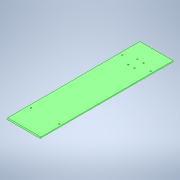
# Autodesk Inventor part: 前カバー中盤
Saved by Autodesk Inventor 2022 (Build 260153000, 153)
## iProperties
Created: 2022-11-07
Part Number: 前カバー中盤
Material: ABS プラスチック
Document SubType Name: Modeling
Designer: tdn82
Density: 1.06 g/cm^3
Appearance: 滑らか - 白
Author: tdn82
Autodesk Inventor part; units mm, degrees
ref_plane "YZ Plane" through (0, 0, 0) normal (1, 0, 0) x (0, 1, 0)
ref_plane "XZ Plane" through (0, 0, 0) normal (0, 1, 0) x (-1, 0, 0)
ref_plane "XY Plane" through (0, 0, 0) normal (0, 0, 1) x (1, 0, 0)
sketch "スケッチ1" plane through (0, 0, 0) normal (0, 1, 0) x (-1, 0, 0)
  line L0 (0, 0) -> (-80, 0)
  line L1 (-80, 0) -> (-80, -320)
  line L2 (-80, -320) -> (0, -320)
  line L3 (0, -320) -> (0, 0)
  dimension "d0" = 320
  dimension "d1" = 80
  constraints: 8 end point, 2 parallel, 1 horizontal, 1 perpendicular
  measures "d0" distance of L2.end L0.start
  measures "d1" distance of L0.start L0.end
extrude "押し出し1" add sketch "スケッチ1" along normal blind 2
sketch "スケッチ3" plane through (0, 0, 0) normal (0, -1, 0) x (1, 0, 0)
  line L0 (80, -320) -> (0, -320) projected
  line L1 (80, 0) -> (80, -320) projected
  point P0 (0, 0)
  point P1 (49, -280)
  point P2 (34, -280)
  point P3 (49, -258)
  point P4 (34, -258)
  dimension "d20" = 40
  dimension "d21" = 31
  dimension "d24" = 15
  dimension "d27" = 22
  constraints: 1 horizontal, 1 vertical, 3 other
  measures "d20" distance from line of L0 point (49, -280)
  measures "d21" distance from line of point (49, -280) L1
  measures "d24" distance of point (49, -280) point (34, -280)
  measures "d27" distance of point (49, -280) point (49, -258)
hole "穴1" at (49, 0, -280) at (34, 0, -280) at (49, 0, -258) at (34, 0, -258) direction (0, 1, 0) diameter 3.2 end through all
chamfer "面取り2" distance 2 angle 45 1 edges at (40, 2, 0)
sketch "スケッチ5" plane through (0, 0, 0) normal (0, -1, 0) x (1, 0, 0)
  line L0 (80, 0) -> (80, -320) projected
  line L1 (0, 0) -> (80, 0) projected
  line L2 (0, -320) -> (0, 0) projected
  point P0 (75, -51)
  point P1 (75, -271)
  point P2 (5, -51)
  point P3 (5, -271)
  dimension "d43" = 5
  dimension "d44" = 51
  dimension "d45" = 220
  dimension "d53" = 5
  dimension "d54" = 51
  dimension "d55" = 220
  dimension "d56" = 5
  measures "d43" distance from line of point (75, -51) L0
  measures "d44" distance from line of point (75, -51) L1
  measures "d45" distance of point (75, -271) point (75, -51)
  measures "d53" distance from line of L2 point (5, -51)
  measures "d54" distance from line of L1 point (5, -51)
  measures "d55" distance of point (5, -51) point (5, -271)
  measures "d56" distance from line of L2 point (5, -271)
hole "穴2" at (75, 0, -51) at (75, 0, -271) at (5, 0, -51) at (5, 0, -271) direction (0, 1, 0) diameter 3.2 end through all
